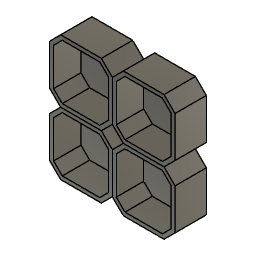
Estanterias-Soporte v1 (Autodesk Fusion 360 design; units mm, degrees)
Autodesk Fusion 360 part; units mm, degrees
sketch "Boceto1" plane through (0, 0, 0) normal (0, 0, 1) x (1, 0, 0)
  line L0 (28.7409, 54.698) -> (428.7409, 54.698)
  line L1 (428.7409, 54.698) -> (428.7409, -345.302)
  line L2 (428.7409, -345.302) -> (28.7409, -345.302)
  line L3 (28.7409, -345.302) -> (28.7409, 54.698)
  dimension "d1" = 400
  dimension "d2" = 400
  constraint horizontal L0
  constraint vertical L1
  constraint horizontal L2
  constraint vertical L3
  measures "d1" distance of L0.start L0.end
  measures "d2" distance of L0.start L2.end
extrude "Extruir1" add sketch "Boceto1" along normal blind 200 makes body 1
chamfer "Chaflán1" distance 70 angle 45 4 edges at (28.7409, 54.698, 100) (428.7409, 54.698, 100) (28.7409, -345.302, 100) (428.7409, -345.302, 100) on bodies 1
move_body "Desplazar1" bodies 1 to x (1, 0, 0) y (0, 0, -1) z (0, 1, 0) at (0, -245.302, 54.698)
shell "Vaciado1" thickness 25 removed faces 1 at (185.4075, -245.302, 133.3333) on bodies 1
copy_body "CopiarPegarCuerpos1" bodies 1 makes body 2
move_body "Desplazar2" bodies 2 to x (1, 0, 0) y (0, 1, 0) z (0, 0, 1) at (0, 0, 400)
copy_body "CopiarPegarCuerpos2" bodies 1 makes body 3
move_body "Desplazar3" bodies 3 to x (1, 0, 0) y (0, 1, 0) z (0, 0, 1) at (400, 0, 0)
copy_body "CopiarPegarCuerpos3" bodies 1 makes body 4
move_body "Desplazar4" bodies 4 to x (1, 0, 0) y (0, 1, 0) z (0, 0, 1) at (400, 0, 400)
